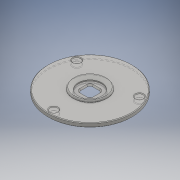
# Autodesk Inventor part: flat_platform_v1_mm
Saved by Autodesk Inventor 2016 (Build 200138000, 138)
## iProperties
Created: 2018-05-30
Part Number: flat_platform_v1_mm
Material: Generic
Document SubType Name: Modeling
Designer: Valued Customer
Density: 1 g/cm^3
Appearance: Default
Author: Valued Customer
Autodesk Inventor part; units mm, degrees
ref_plane "YZ Plane" through (0, 0, 0) normal (1, 0, 0) x (0, 1, 0)
ref_plane "XZ Plane" through (0, 0, 0) normal (0, 1, 0) x (-1, 0, 0)
sketch "Main Platform" plane through (0, 0, 0) normal (0, 1, 0) x (-1, 0, 0)
  circle A0 centre (0, 0) radius 36
  dimension "d0" = 72
  constraints: 1 centre point, 1 coincident
  measures "d0" diameter of A0
extrude "Main Platform Extrusion" add sketch "Main Platform" along normal blind 5
sketch "Main Hole" plane through (0, 0, 0) normal (0, -1, 0) x (1, 0, 0)
  circle A0 centre (0, 0) radius 36 construction
  circle A1 centre (0, 0) radius 10
  dimension "d3" = 20
  constraints: 1 centre point, 1 coincident
  measures "d3" diameter of A1
extrude "Main Hole Cutout" cut sketch "Main Hole" against normal through all
sketch "Bottom Magnet Holes (MASTER)" plane through (0, 0, 0) normal (0, -1, 0) x (1, 0, 0)
  circle A0 centre (0, 0) radius 10 construction
  circle A1 centre (0, 0) radius 36 construction
  circle A2 centre (0, 0) radius 36 construction
  line L0 (0, -50.4) -> (0, 50.4) construction
  line L1 (0, 36) -> (0, -36) construction
  circle A3 centre (0, 0) radius 31 construction
  line L2 (0, 0) -> (26.8468, 15.5) construction
  line L3 (0, 0) -> (-26.8468, 15.5) construction
  line L4 (0, 0) -> (0, -31) construction
  dimension "d37" = 5
  dimension "d38" = 120
  dimension "d39" = 120
  constraints: 8 end point, 5 point on circle, 4 coincident, 3 point on line, 1 centre point
  measures "d37" radial gap between concentric circles of A1 A3
  measures "d38" angle of L0 L2
  measures "d39" angle of L3 L0
chamfer "Saline Well" distance 3.5 angle 30 1 edges at (-10, 5, 0) measured on face at (-27.0099, 5, -2.7674)
sketch "Top Magnet Holes" plane through (0, 5, 0) normal (0, 1, 0) x (1, 0, 0)
  circle A0 centre (0, 0) radius 31 construction
  point P0 (26.8468, -15.5)
  point P1 (-26.8468, -15.5)
  point P2 (0, 31)
ref_plane "Shim Holder Plane" through (0, 1, 0) normal (0, -1, 0) x (1, 0, 0)
sketch "Shim Holder" plane through (0, 1, 0) normal (0, -1, 0) x (1, 0, 0)
  circle A0 centre (0, 0) radius 36 construction
  circle A1 centre (0, 0) radius 13.5 construction
  circle A2 centre (0, 0) radius 15
  dimension "d137" = 30
  constraints: 1 centre point, 1 coincident
  measures "d137" diameter of A2
extrude "Shim Holder Extrusion" add sketch "Shim Holder" against normal blind 1
sketch "Sketch22" plane through (0, 5, 0) normal (0, 1, 0) x (1, 0, 0)
  circle A0 centre (0, 0) radius 36 construction
  circle A1 centre (0, 0) radius 13.5 construction
  circle A2 centre (0, 0) radius 14.5
  circle A3 centre (0, 0) radius 36
  dimension "d110" = 1
  constraints: 2 centre point, 2 coincident, 1 concentric
  measures "d110" radial gap between concentric circles of A1 A2
extrude "Saline Well Recess" cut sketch "Sketch22" against normal blind 1.5
fillet "Fillet4" radius 1.5 1 edges at (-14.5, 5, 0)
hole "Top Magnet Recess" at (26.8468, 5, 15.5) at (0, 5, -31) at (-26.8468, 5, 15.5) direction (0, -1, 0) diameter 6.5 depth 2
hole "Bottom Magnet Recess" at (26.8468, 0, 15.5) at (0, 0, -31) at (-26.8468, 0, 15.5) direction (0, 1, 0) diameter 6.5 depth 0.5
chamfer "Chamfer6" distance 0.5 angle 45 9 edges at (36, 0, 0) (0, 0, -27.75) (26.8468, 0, 18.75) (-26.8468, 0, 18.75) (36, 3.5, 0) (-26.8468, 3.5, 12.25) (26.8468, 3.5, 12.25) (0, 3.5, -34.25) (-10, 0, 0)
sketch "Sketch25" plane through (0, 1, 0) normal (0, -1, 0) x (1, 0, 0)
  line L0 (-3, 5) -> (3, 5)
  line L1 (5, 3) -> (5, -3)
  line L2 (3, -5) -> (-3, -5)
  line L3 (-5, -3) -> (-5, 3)
  line L4 (-5, 5) -> (5, -5) construction
  line L5 (5, 5) -> (-5, -5) construction
  arc A0 (3, -5) -> (5, -3) centre (3, -3) ccw
  arc A1 (-5, -3) -> (-3, -5) centre (-3, -3) ccw
  arc A2 (-3, 5) -> (-5, 3) centre (-3, 3) ccw
  arc A3 (5, 3) -> (3, 5) centre (3, 3) ccw
  point P0 (0, 0)
  point P1 (0, 0)
  dimension "d140" = 10
  dimension "d141" = 10
  dimension "d142" = 2
  constraints: 12 end point, 8 point on circle, 8 point on line, 8 tangent, 4 centre point, 3 equal radius, 2 midpoint, 2 parallel, 1 coincident, 1 horizontal, 1 perpendicular
  measures "d140" distance of L5.start L4.end
  measures "d141" distance of L4.start L5.start
  measures "d142" radius of A0
extrude "Extrusion14" cut sketch "Sketch25" against normal through all
chamfer "Chamfer9" distance 1 angle 45 8 edges at (5, 2, 0) (4.4142, 2, 4.4142) (0, 2, 5) (-4.4142, 2, 4.4142) (-5, 2, 0) (-4.4142, 2, -4.4142) (0, 2, -5) (4.4142, 2, -4.4142)
body "Solid1"
